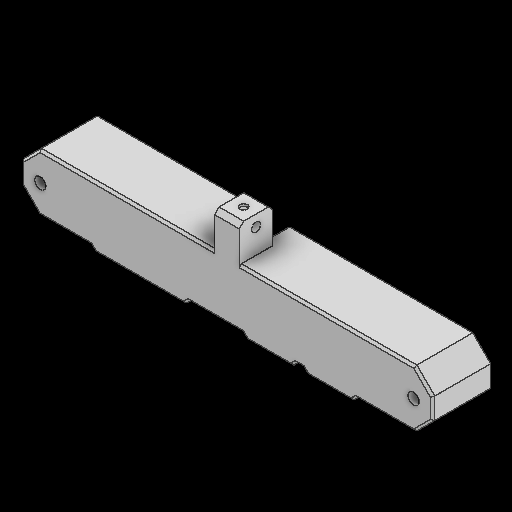
# Autodesk Inventor part: DepthCameraHousing2
Saved by Autodesk Inventor 2025.2 (Build 292293000, 293)
## iProperties
Created: 2026-02-04
Part Number: DepthCameraHousing2
Material: Generic
Document SubType Name: Modeling
Designer: valer
Density: 1 g/cm^3
Appearance: Default
Author: valer
Autodesk Inventor part; units mm, degrees
ref_plane "YZ Plane" through (0, 0, 0) normal (1, 0, 0) x (0, 1, 0)
ref_plane "XZ Plane" through (0, 0, 0) normal (0, 1, 0) x (-1, 0, 0)
ref_plane "XY Plane" through (0, 0, 0) normal (0, 0, 1) x (1, 0, 0)
sketch "Base" plane through (0, 0, 0) normal (0, 0, 1) x (1, 0, 0)
  line L0 (-82, 10.75) -> (82, 10.75)
  line L1 (82, 10.75) -> (82, -10.75)
  line L2 (82, -10.75) -> (-82, -10.75)
  line L3 (-82, -10.75) -> (-82, 10.75)
  line L4 (-82, 10.75) -> (82, -10.75) construction
  line L5 (82, 10.75) -> (-82, -10.75) construction
  line L6 (-123.2, 0) -> (123.2, 0) construction
  line L7 (0, -17.85) -> (0, 17.85) construction
  line L8 (84, 12.75) -> (-84, 12.75)
  line L9 (-84, 12.75) -> (-84, -12.75)
  line L10 (-84, -12.75) -> (84, -12.75)
  line L11 (84, -12.75) -> (84, 12.75)
  circle A0 centre (-83.5, 0) radius 4.5
  circle A1 centre (83.5, 0) radius 4.5
  line L12 (-83.5, 0) -> (83.5, 0) construction
  circle A2 centre (-83.5, 0) radius 1
  circle A3 centre (83.5, 0) radius 1
  point P0 (0, 0)
  point P1 (-84, 4.4721)
  point P2 (-84, -4.4721)
  point P3 (84, -4.4721)
  point P4 (84, 4.4721)
  point P5 (-82, 4.2426)
  point P6 (82, 4.2426)
  point P7 (82, -4.2426)
  point P8 (-82, -4.2426)
  dimension "d0" = 21.5
  dimension "d14" = 2
  dimension "d51" = 9
  dimension "d52" = 167
  dimension "d53" = 164
  dimension "d54" = 2
  dimension "d55" = 2
  constraints: 22 end point, 4 centre point, 4 parallel, 3 midpoint, 2 coincident, 2 perpendicular, 2 point on line, 1 collinear, 1 equal radius, 1 horizontal, 3 other
  measures "d0" distance between parallel lines of L2 L0
  measures "d14" distance between parallel lines of L0 L8
  measures "d51" diameter of A0
  measures "d52" distance of L12.end L12.start
  measures "d53" distance between parallel lines of L1 L3
  measures "d54" diameter of A2
  measures "d55" diameter of A3
extrude "BaseFeature" add sketch "Base" along normal blind 23 contours L3 A0 L9 L8 L11 A1 L1 L0 | A0 L3 | L3 A0 L9 A2 | A1 L11 A3 L1 | L1 A1 | L3 L2 L1 A1 L11 L10 L9 A0 | L9 A2 A0 | A1 L11 A3
extrude "BackFeature" add sketch "Base" against normal blind 3 contours L3 A0 L9 L8 L11 A1 L1 L0 | L0 L1 A1 L2 L3 A0 | A0 L3 | L3 A0 L9 A2 | A1 L11 A3 L1 | L1 A1 | L3 L2 L1 A1 L11 L10 L9 A0 | L9 A2 A0 | A1 L11 A3
sketch "Mount" plane through (0, 0, -3) normal (0, 0, -1) x (-1, 0, 0)
  line L0 (126, 0) -> (-126, 0) construction
  line L1 (0, -19.25) -> (0, 19.25) construction
  line L2 (84, 12.75) -> (-84, 12.75) projected
  line L3 (5.5, 12.75) -> (2.75, 12.75)
  line L4 (5.5, 28.75) -> (5.5, 12.75)
  line L5 (-5.5, 28.75) -> (-5.5, 12.75)
  line L6 (5.5, 28.75) -> (-5.5, 28.75)
  point P0 (0, 0)
  point P1 (-5.5, 12.75)
  dimension "d70" = 16
  dimension "d121" = 11
  constraints: 12 end point, 3 horizontal, 2 symmetric about line, 1 point on line, 1 vertical, 4 other
  measures "d70" distance of L4.start L3.start
  measures "d121" distance between parallel lines of L5 L4
extrude "MountFeature" add sketch "Mount" against normal blind 15
chamfer "MountChamferFeature" distance 2 angle 45 2 edges at (0, 28.75, -3) (0, 28.75, 12)
sketch "Sides" plane through (0, 0, -3) normal (0, 0, -1) x (-1, 0, 0)
  line L0 (0, -21.05) -> (0, 37.05) construction
  line L1 (-84, -12.75) -> (84, -12.75) projected
  line L2 (-84, -12.75) -> (-92, -4.75)
  line L3 (128.8, 0) -> (-128.8, 0) construction
  line L4 (-92, -4.75) -> (-92, 0)
  arc A0 (-77.585, 12.415) -> (-77.585, -12.415) centre (-77.585, 0) ccw construction
  arc A1 (-84, 4.4721) -> (-84, -4.4721) centre (-83.5, 0) ccw projected
  line L5 (84, -12.75) -> (92, -4.75)
  line L6 (92, -4.75) -> (92, 0)
  line L7 (-84, 12.75) -> (-92, 4.75)
  line L8 (-92, 4.75) -> (-92, 0)
  line L9 (84, 12.75) -> (92, 4.75)
  line L10 (92, 4.75) -> (92, 0)
  line L11 (84, -12.75) -> (84, -4.4721) projected
  arc A2 (84, -4.4721) -> (84, 4.4721) centre (83.5, 0) ccw projected
  line L12 (84, 4.4721) -> (84, 12.75) projected
  line L13 (-84, -4.4721) -> (-84, -12.75) projected
  line L14 (-84, 12.75) -> (-84, 4.4721) projected
  point P0 (0, 0)
  point P1 (-88, 0)
  dimension "d76" = 4
  dimension "d77" = 45
  constraints: 16 end point, 6 symmetric about line, 1 perpendicular, 1 point on circle, 1 point on line
  measures "d76" distance of L4.end point (-88, 0)
  measures "d77" angle of L2 L3
extrude "SidesFeature" add sketch "Sides" against normal up to surface (26 mm away)
sketch "Decorative" plane through (0, 0, 23) normal (0, 0, 1) x (1, 0, 0)
  line L0 (-84, -12.75) -> (84, -12.75) projected
  line L1 (58, -12.75) -> (56, -14.75)
  line L2 (56, -14.75) -> (36, -14.75)
  line L3 (36, -14.75) -> (34, -12.75)
  circle A0 centre (46, 0) radius 9.875 construction
  line L4 (46, -14.75) -> (46, 0) construction
  circle A1 centre (19, 0) radius 9.875 construction
  line L5 (31, -12.75) -> (29, -14.75)
  line L6 (29, -14.75) -> (9, -14.75)
  line L7 (9, -14.75) -> (7, -12.75)
  line L8 (19, -14.75) -> (19, 0) construction
  line L9 (-17, -12.75) -> (-19, -14.75)
  line L10 (-19, -14.75) -> (-59, -14.75)
  line L11 (-59, -14.75) -> (-61, -12.75)
  point P0 (0, 0)
  dimension "d80" = 45
  dimension "d81" = 45
  dimension "d82" = 2
  dimension "d83" = 20
  dimension "d84" = 45
  dimension "d85" = 45
  dimension "d86" = 40
  dimension "d89" = 45
  dimension "d90" = 45
  dimension "d91" = 24
  constraints: 22 end point, 6 point on line, 3 collinear, 2 midpoint, 2 perpendicular, 1 horizontal, 1 parallel, 1 vertical
  measures "d80" angle of L0 L3
  measures "d81" angle of L0 L1
  measures "d82" distance between parallel lines of L0 L2
  measures "d83" distance of L1.end L2.end
  measures "d84" angle of L0 L5
  measures "d85" angle of L0 L7
  measures "d86" distance of L9.end L10.end
  measures "d89" angle of L0 L9
  measures "d90" angle of L0 L11
  measures "d91" distance of L9.start L7.end
extrude "DecorativeFeature" add sketch "Decorative" against normal up to surface (26 mm away)
chamfer "BackChamferFeature" distance 1 angle 45 21 edges at (-72.5, -12.75, -3) (-88, -8.75, -3) (-92, 0, -3) (-88, 8.75, -3) (-44.75, 12.75, -3) (-60, -13.75, -3) (-39, -14.75, -3) (-18, -13.75, -3) (-5, -12.75, -3) (8, -13.75, -3) (19, -14.75, -3) (30, -13.75, -3) (32.5, -12.75, -3) (35, -13.75, -3) (46, -14.75, -3) (57, -13.75, -3) (71, -12.75, -3) (88, -8.75, -3) (92, 0, -3) (88, 8.75, -3) (44.75, 12.75, -3)
sketch "MountHole" plane through (5.5, 12.75, 12) normal (1, 0, 0) x (0, 0, -1)
  line L0 (13, 16) -> (2, 16) projected
  line L1 (7.5, 16) -> (7.5, 11) construction
  circle A0 centre (7.5, 11) radius 2
  point P0 (12, -12.75)
  point P1 (15, 16)
  point P2 (0, 16)
  dimension "d97" = 4
  dimension "d98" = 5
  constraints: 2 end point, 1 centre point, 1 coincident, 1 midpoint, 1 vertical
  measures "d97" diameter of A0
  measures "d98" distance of L1.start L1.end
extrude "MountHoleFeature" cut sketch "MountHole" along normal through all both and the other way through all
sketch "DecorativeHoles" plane through (36, -14.75, 23) normal (0, -1, 0) x (1, 0, 0)
  line L0 (20, -25) -> (0, -25) construction
  line L1 (20, 0) -> (20, -25) construction
  line L2 (0, 0) -> (20, 0) construction
  line L3 (0, 0) -> (0, -25) construction
  line L4 (-7, -25) -> (-27, -25) construction
  line L5 (-7, 0) -> (-7, -25) construction
  line L6 (-27, 0) -> (-7, 0) construction
  line L7 (-27, 0) -> (-27, -25) construction
  line L8 (-55, -25) -> (-95, -25) construction
  line L9 (-55, 0) -> (-55, -25) construction
  line L10 (-95, 0) -> (-55, 0) construction
  line L11 (-95, 0) -> (-95, -25) construction
  line L12 (16, -7) -> (4, -19) construction
  line L13 (15.1868, -6.1868) -> (3.1868, -18.1868)
  line L14 (4.8132, -19.8132) -> (16.8132, -7.8132)
  arc A0 (16.8132, -7.8132) -> (15.1868, -6.1868) centre (16, -7) ccw
  arc A1 (3.1868, -18.1868) -> (4.8132, -19.8132) centre (4, -19) ccw
  line L15 (20, -19) -> (0, -19) construction
  line L16 (20, -4) -> (0, -4) construction
  line L17 (14.5858, -19) -> (16, -17.5858) construction
  line L18 (13.7726, -18.1868) -> (15.1868, -16.7726)
  line L19 (16.8132, -18.399) -> (15.399, -19.8132)
  arc A2 (13.7726, -18.1868) -> (15.399, -19.8132) centre (14.5858, -19) ccw
  arc A3 (16.8132, -18.399) -> (15.1868, -16.7726) centre (16, -17.5858) ccw
  line L20 (4, -8.4142) -> (5.4142, -7) construction
  line L21 (4.8132, -9.2274) -> (6.2274, -7.8132)
  line L22 (4.601, -6.1868) -> (3.1868, -7.601)
  arc A4 (3.1868, -7.601) -> (4.8132, -9.2274) centre (4, -8.4142) ccw
  arc A5 (6.2274, -7.8132) -> (4.601, -6.1868) centre (5.4142, -7) ccw
  line L23 (9.2929, -19) -> (16, -12.2929) construction
  line L24 (10.1061, -19.8132) -> (16.8132, -13.1061)
  line L25 (15.1868, -11.4797) -> (8.4797, -18.1868)
  arc A6 (8.4797, -18.1868) -> (10.1061, -19.8132) centre (9.2929, -19) ccw
  arc A7 (16.8132, -13.1061) -> (15.1868, -11.4797) centre (16, -12.2929) ccw
  line L26 (4, -13.7071) -> (10.7071, -7) construction
  line L27 (3.1868, -12.8939) -> (9.8939, -6.1868)
  line L28 (11.5203, -7.8132) -> (4.8132, -14.5203)
  arc A8 (3.1868, -12.8939) -> (4.8132, -14.5203) centre (4, -13.7071) ccw
  arc A9 (11.5203, -7.8132) -> (9.8939, -6.1868) centre (10.7071, -7) ccw
  line L29 (20, -19) -> (0, -4) construction
  line L30 (-2, -25) -> (-5, -25) projected
  line L31 (-5, 0) -> (-2, 0) projected
  line L32 (-10.1868, -18.399) -> (-11.601, -19.8132)
  arc A10 (-13.2274, -18.1868) -> (-11.601, -19.8132) centre (-12.4142, -19) ccw
  arc A11 (-10.1868, -18.399) -> (-11.8132, -16.7726) centre (-11, -17.5858) ccw
  line L33 (-13.2274, -18.1868) -> (-11.8132, -16.7726)
  line L34 (-16.8939, -19.8132) -> (-10.1868, -13.1061)
  arc A12 (-18.5203, -18.1868) -> (-16.8939, -19.8132) centre (-17.7071, -19) ccw
  line L35 (-11.8132, -11.4797) -> (-18.5203, -18.1868)
  arc A13 (-10.1868, -13.1061) -> (-11.8132, -11.4797) centre (-11, -12.2929) ccw
  line L36 (-22.1868, -19.8132) -> (-10.1868, -7.8132)
  arc A14 (-10.1868, -7.8132) -> (-11.8132, -6.1868) centre (-11, -7) ccw
  line L37 (-11.8132, -6.1868) -> (-23.8132, -18.1868)
  arc A15 (-23.8132, -18.1868) -> (-22.1868, -19.8132) centre (-23, -19) ccw
  arc A16 (-23.8132, -12.8939) -> (-22.1868, -14.5203) centre (-23, -13.7071) ccw
  line L38 (-15.4797, -7.8132) -> (-22.1868, -14.5203)
  line L39 (-23.8132, -12.8939) -> (-17.1061, -6.1868)
  arc A17 (-15.4797, -7.8132) -> (-17.1061, -6.1868) centre (-16.2929, -7) ccw
  arc A18 (-20.7726, -7.8132) -> (-22.399, -6.1868) centre (-21.5858, -7) ccw
  line L40 (-22.1868, -9.2274) -> (-20.7726, -7.8132)
  line L41 (-22.399, -6.1868) -> (-23.8132, -7.601)
  arc A19 (-23.8132, -7.601) -> (-22.1868, -9.2274) centre (-23, -8.4142) ccw
  point P0 (-36, -23)
  point P1 (10, -13)
  point P2 (15.2929, -18.2929)
  point P3 (12.6464, -15.6464)
  point P4 (4.7071, -7.7071)
  dimension "d102" = 45
  dimension "d104" = 4
  dimension "d105" = 4
  dimension "d106" = 4
  dimension "d107" = 4
  dimension "d108" = 3.7426
  dimension "d109" = 3.7426
  dimension "d110" = 3.7426
  dimension "d111" = 3.7426
  dimension "d113" = 4
  dimension "d114" = 4
  dimension "d115" = 4
  dimension "d118" = 6
  dimension "d119" = 2
  dimension "d120" = 1.15
  dimension "d124" = 27
  constraints: 66 end point, 40 point on circle, 20 centre point, 12 symmetric about line, 12 tangent, 7 point on line, 5 parallel, 4 midpoint, 2 equal radius, 2 perpendicular, 1 horizontal, 54 other
  measures "d102" angle of L12 L1
  measures "d104" distance from line of L1 L12.start
  measures "d105" distance between parallel lines of L2 L16
  measures "d106" distance from line of L1 L17.end
  measures "d107" distance from line of L1 L23.end
  measures "d108" distance between parallel lines of L23 L17
  measures "d109" distance between parallel lines of L12 L23
  measures "d110" distance between parallel lines of L26 L12
  measures "d111" distance from line of point (4.707, -7.707) L26
  measures "d113" distance from line of L3 L20.start
  measures "d114" distance from line of L3 L12.end
  measures "d115" distance from line of L3 L26.start
  measures "d118" distance between parallel lines of L0 L15
  measures "d119" distance of L17.start L17.end
  measures "d120" radius of A1
  measures "d124" distance of L19.start L32.start
extrude "DecorativeHolesFeature" cut sketch "DecorativeHoles" against normal up to surface (4 mm away)
sketch "OneMoreDecorativeHole" plane through (-59, -14.75, 23) normal (0, -1, 0) x (1, 0, 0)
  line L0 (34, -4) -> (6, -21) construction
  line L1 (33.4032, -3.017) -> (5.4032, -20.017)
  line L2 (6.5968, -21.983) -> (34.5968, -4.983)
  arc A0 (34.5968, -4.983) -> (33.4032, -3.017) centre (34, -4) ccw
  arc A1 (5.4032, -20.017) -> (6.5968, -21.983) centre (6, -21) ccw
  arc A2 (71.1868, -18.1868) -> (72.8132, -19.8132) centre (72, -19) ccw projected
  line L3 (0, 0) -> (40, 0) projected
  line L4 (40, 0) -> (40, -25) projected
  line L5 (0, 0) -> (0, -25) projected
  line L6 (40, -25) -> (0, -25) projected
  point P0 (59, -23)
  point P1 (20, -12.5)
  dimension "d132" = 4
  dimension "d133" = 6
  dimension "d134" = 6
  dimension "d135" = 4
  constraints: 8 end point, 4 point on circle, 4 tangent, 2 centre point, 1 equal radius, 1 midpoint, 1 parallel
  measures "d132" distance from line of L3 L0.start
  measures "d133" distance from line of L4 L0.start
  measures "d134" distance from line of L5 L0.end
  measures "d135" distance from line of L6 L0.end
chamfer "FrontChamferFeature" distance 4 angle 45 1 edges at (0, 12.75, 12)
extrude "OneMoreDecorativeHoleFeature" cut sketch "OneMoreDecorativeHole" against normal up to surface (4 mm away) contours A0 L2 A1 L1
fillet "InsideFilletsFeature" radius 0.5 16 edges at (82, -10.75, 11.5) (82, -4.2426, 11.5) (82, 4.2426, 11.5) (82, 10.75, 11.5) (0, 10.75, 0) (82, 7.4963, 0) (79, 0, 0) (82, -7.4963, 0) (0, -10.75, 0) (-82, -7.4963, 0) (-79, 0, 0) (-82, -4.2426, 11.5) (-82, 4.2426, 11.5) (-82, 7.4963, 0) (-82, 10.75, 11.5) (-82, -10.75, 11.5)
sketch "SnapFitHolesBottom" plane through (5.25, -10.75, -2) normal (0, 1, 0) x (1, 0, 0)
  line L0 (76.25, -25) -> (-86.75, -25) projected
  line L1 (66.7, -25) -> (40.2, -25)
  line L2 (40.2, -25) -> (40.2, -23)
  line L3 (40.2, -23) -> (66.7, -23)
  line L4 (66.7, -23) -> (66.7, -25)
  line L5 (-86.75, -25) -> (76.25, -25) projected
  line L6 (23.7, -25) -> (15.2, -25)
  line L7 (15.2, -25) -> (15.2, -23)
  line L8 (15.2, -23) -> (23.7, -23)
  line L9 (23.7, -23) -> (23.7, -25)
  line L10 (-2.4236, -25) -> (-8.9236, -25)
  line L11 (-8.9236, -25) -> (-8.9236, -23)
  line L12 (-8.9236, -23) -> (-2.4236, -23)
  line L13 (-2.4236, -23) -> (-2.4236, -25)
  line L14 (-25.75, -25) -> (-34.75, -25)
  line L15 (-34.75, -25) -> (-34.75, -23)
  line L16 (-34.75, -23) -> (-25.75, -23)
  line L17 (-25.75, -23) -> (-25.75, -25)
  line L18 (-51.75, -25) -> (-77.75, -25)
  line L19 (-77.75, -25) -> (-77.75, -23)
  line L20 (-77.75, -23) -> (-51.75, -23)
  line L21 (-51.75, -23) -> (-51.75, -25)
  line L22 (-5.25, 7.8) -> (-5.25, -39.8) construction
  point P0 (-5.25, -2)
  point P1 (-10.75, -33)
  point P2 (-5.25, -25)
  point P3 (19.45, -23)
  point P4 (53.45, -23)
  point P5 (-30.25, -23)
  point P6 (-64.75, -23)
  point P7 (40.2, -25)
  point P8 (15.2, -25)
  point P9 (-8.9236, -25)
  point P10 (-2.4236, -25)
  point P11 (-34.75, -25)
  point P12 (-77.75, -25)
  point P13 (-51.75, -25)
  dimension "d202" = 26.5
  dimension "d203" = 8.5
  dimension "d204" = 6.5
  dimension "d205" = 9
  dimension "d206" = 26
  dimension "d207" = 2
  dimension "d208" = 24.7
  dimension "d209" = 34
  dimension "d210" = 25
  dimension "d211" = 59.5
  constraints: 40 end point, 10 parallel, 5 horizontal, 5 perpendicular, 4 collinear, 4 midpoint, 4 point on line, 5 other
  measures "d202" distance of L2.end L3.end
  measures "d203" distance of L7.end L8.end
  measures "d204" distance of L11.end L12.end
  measures "d205" distance of L15.end L16.end
  measures "d206" distance of L19.end L20.end
  measures "d207" distance of L3.end L1.start
  measures "d208" distance from line of point (19.45, -23) L22
  measures "d209" distance of point (53.45, -23) point (19.45, -23)
  measures "d210" distance from line of point (-30.25, -23) L22
  measures "d211" distance from line of L22 point (-64.75, -23)
sketch "SnapFitHolesTop" plane through (-59.25, 10.75, 22.5) normal (0, -1, 0) x (1, 0, 0)
  line L0 (140.75, 0.5) -> (-22.25, 0.5) projected
  line L1 (-13.75, 0.5) -> (-2.75, 0.5)
  line L2 (-2.75, 0.5) -> (-2.75, -1.5)
  line L3 (-2.75, -1.5) -> (-13.75, -1.5)
  line L4 (-13.75, -1.5) -> (-13.75, 0.5)
  line L5 (13.1, 0.5) -> (-1.75, 0.5)
  line L6 (-1.75, 0.5) -> (-1.75, -1.5)
  line L7 (-1.75, -1.5) -> (13.1, -1.5)
  line L8 (13.1, -1.5) -> (13.1, 0.5)
  line L9 (45.6, 0.5) -> (50.6, 0.5)
  line L10 (50.6, 0.5) -> (50.6, -1.5)
  line L11 (50.6, -1.5) -> (45.6, -1.5)
  line L12 (45.6, -1.5) -> (45.6, 0.5)
  line L13 (52.6, 0.5) -> (61.25, 0.5)
  line L14 (61.25, 0.5) -> (61.25, -1.5)
  line L15 (61.25, -1.5) -> (52.6, -1.5)
  line L16 (52.6, -1.5) -> (52.6, 0.5)
  line L17 (68.25, 0.5) -> (68.25, -24.5) projected
  line L18 (68.25, 0.5) -> (74.25, 0.5)
  line L19 (74.25, 0.5) -> (74.25, -1.5)
  line L20 (74.25, -1.5) -> (68.25, -1.5)
  line L21 (68.25, -1.5) -> (68.25, 0.5)
  line L22 (104.75, 0.5) -> (132.75, 0.5)
  line L23 (132.75, 0.5) -> (132.75, -1.5)
  line L24 (132.75, -1.5) -> (104.75, -1.5)
  line L25 (104.75, -1.5) -> (104.75, 0.5)
  line L26 (59.25, -30.7) -> (59.25, 5.7) construction
  line L27 (-1.75, -24.5) -> (-1.75, 0.5) projected
  point P0 (59.25, -22.5)
  point P1 (-1.75, 0.5)
  point P2 (68.25, -1.5)
  dimension "d212" = 2
  dimension "d213" = 2
  dimension "d214" = 6
  dimension "d215" = 28
  dimension "d216" = 30.5
  dimension "d217" = 2
  dimension "d218" = 5
  dimension "d219" = 8.65
  dimension "d220" = 32.5
  dimension "d221" = 1
  dimension "d222" = 11
  constraints: 48 end point, 12 parallel, 6 collinear, 6 horizontal, 6 perpendicular, 6 other
  measures "d212" distance of L3.end L1.start
  measures "d213" distance from line of L14.end L26
  measures "d214" distance of L19.end L20.end
  measures "d215" distance of L23.end L24.end
  measures "d216" distance of L24.end L19.end
  measures "d217" distance of L15.end L10.end
  measures "d218" distance of L10.end L11.end
  measures "d219" distance from line of L26 L10.end
  measures "d220" distance of L11.end L7.end
  measures "d221" distance of L6.end L2.end
  measures "d222" distance of L2.end L3.end
extrude "SnapFitHolesBottomFeature" cut sketch "SnapFitHolesBottom" against normal blind 0.75
extrude "SnapFitHolesTopFeature" cut sketch "SnapFitHolesTop" against normal blind 0.75
sketch "Countersinks" plane through (0, 0, -3) normal (0, 0, -1) x (-1, 0, 0)
  circle A0 centre (83.5, 0) radius 1 projected
  circle A1 centre (-83.5, 0) radius 1 projected
  circle A2 centre (83.5, 0) radius 2.5
  circle A3 centre (-83.5, 0) radius 2.5
  point P0 (0, 0)
  dimension "d229" = 5
  constraints: 2 centre point, 2 coincident, 1 equal radius
  measures "d229" diameter of A2
extrude "CountersinksFeature" cut sketch "Countersinks" against normal blind 20 contours A0 | A1 | A2 | A3
sketch "CenterIndicator" plane through (-5.5, 28.75, 10) normal (0, 1, 0) x (1, 0, 0)
  line L0 (11, 0) -> (0, 0) projected
  line L1 (0, 11) -> (11, 11) projected
  line L2 (11, 0) -> (0, 11) construction
  circle A0 centre (5.5, 5.5) radius 1.75
  point P0 (5.5, 10)
  dimension "d234" = 3.5
  constraints: 2 end point, 1 centre point, 1 midpoint
  measures "d234" diameter of A0
extrude "CenterIndicatorFeature" cut sketch "CenterIndicator" against normal blind 1
mirror "Mirror1" about plane through (0, 0, 0) normal (0, 0, 1) remove original yes
delete faces "Delete4" heal yes whole lump no faces at (-61, 11, -22.3333)
delete faces "Delete5" heal yes whole lump no faces at (1.8333, 15.4167, -13.3333)
sketch "CableGland" plane through (-84, 12.75, -23) normal (0, 1, 0) x (1, 0, 0)
  line L0 (77.35, -2) -> (77.35, 0) projected
  line L1 (86, 0) -> (86, -2) projected
  line L2 (86, -2) -> (77.35, -2) projected
  line L3 (77.35, -2) -> (77.35, -11)
  line L4 (86, -2) -> (86, -11)
  line L5 (86, -11) -> (77.35, -11)
  line L6 (81.675, -11) -> (81.675, -8) construction
  line L7 (168, 0) -> (0, 0) projected
  line L8 (78.5, -26) -> (0.4142, -26) projected
  line L9 (89.5, -11) -> (78.5, -11) projected
  point P0 (84, -23)
  constraints: 8 end point, 3 vertical, 1 collinear, 1 midpoint, 1 perpendicular
extrude "CableGlandFeature" cut sketch "CableGland" against normal up to surface (2 mm away)
fillet "Fillet4" radius 2 2 edges at (-6.65, 11.75, -12) (2, 11.75, -12)
equation "\"d81\" = d80"
equation "\"d84\" = d80"
equation "\"d89\" = d80"
equation "\"d90\" = d80"
equation "\"d104\" = d103"
equation "\"d105\" = d103"
equation "\"d106\" = d103"
equation "\"d107\" = d104"
equation "\"d109\" = d108"
equation "\"d110\" = d108"
equation "\"d111\" = d108"
equation "\"d103\" = 4"
body "Solid1"
